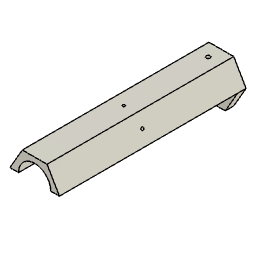
TwoPartTubeJigLong (Autodesk Fusion 360 design; units mm, degrees)
Autodesk Fusion 360 part; units mm, degrees
sketch "Sketch1" plane through (0, 0, 0) normal (0, 1, 0) x (1, 0, 0)
  circle A0 centre (0, 0) radius 9.525
  line L0 (-7.3323, -12.7) -> (7.3323, -12.7)
  line L1 (7.3323, -12.7) -> (14.6647, 0)
  line L2 (14.6647, 0) -> (7.3323, 12.7)
  line L3 (7.3323, 12.7) -> (-7.3323, 12.7)
  line L4 (-7.3323, 12.7) -> (-14.6647, 0)
  line L5 (-14.6647, 0) -> (-7.3323, -12.7)
  dimension "d1" = 19.05
  dimension "d2" = 25.4
  constraint coincident A0.centre origin
  constraint horizontal L0
  measures "d1" diameter of A0
  measures "d2" distance of L0 L3
extrude "Extrude1" add sketch "Sketch1" along normal mid plane 105.6 makes body 1
sketch "Sketch2" plane through (0, 0, 0) normal (0, 0, 1) x (1, 0, 0)
hole "Hole1" at (0, 0, 0) direction (0, 0, -1) diameter 1.588 end through all bodies 1
pattern_circular "C-Pattern1" count 6 over 360 about axis through (0, 1.75, 0) along (0, 1, 0) of "Hole1"
split "Split1" by plane through (0, 0, 0) normal (0, 0, 1) bodies 1 makes body 2 at (9.5132, 17.6, 0.4748)
sketch "Sketch3" plane through (0, 52.8, 0) normal (0, 1, 0) x (-1, 0, 0)
  line L0 (-9.525, 0) -> (-14.6647, 0)
  line L1 (-14.6647, 0) -> (-7.3323, -12.7)
  line L2 (-7.3323, -12.7) -> (7.3323, -12.7)
  line L3 (7.3323, -12.7) -> (14.6647, 0)
  line L4 (14.6647, 0) -> (9.525, 0)
  arc A0 (-9.525, 0) -> (9.525, 0) centre (0, 0) ccw
  line L5 (-14.6647, 0) -> (-9.525, 0)
  arc A1 (9.525, 0) -> (-9.525, 0) centre (0, 0) ccw
  line L6 (9.525, 0) -> (14.6647, 0)
  line L7 (14.6647, 0) -> (7.3323, 12.7)
  line L8 (7.3323, 12.7) -> (-7.3323, 12.7)
  line L9 (-7.3323, 12.7) -> (-14.6647, 0)
extrude "Extrude2" add sketch "Sketch3" 2 faces at (-0.2373, 52.8, -11.6328) (-10.1929, 52.8, 5.6109) along normal blind 5 separate body on bodies 1 2 makes body 3
combine "Combine1" operation add target body 3 tool bodies 2
sketch "Sketch4" plane through (0, 0, -12.7) normal (0, 0, -1) x (1, 0, 0)
  circle A0 centre (0, 0) radius 0.794
  line L0 (-7.3323, 52.8) -> (-7.3323, -52.8)
  line L1 (-7.3323, -52.8) -> (7.3323, -52.8)
  line L2 (7.3323, -52.8) -> (7.3323, 52.8)
  line L3 (7.3323, 52.8) -> (-7.3323, 52.8)
  point P0 (0, -50.06)
  dimension "d12" = 2.74
  measures "d12" distance of L1 P0
hole "Hole2" at (0, 50.06, -12.7) direction (0, 0, 1) diameter 2.3813 end through all bodies 3 1
hidden bodies 1
equation "d12 = 0.061 in + 3 in / 64"
equation "d14 = 3 in / 32"
